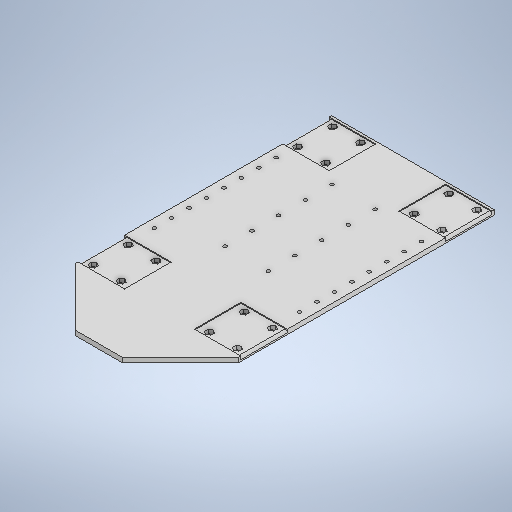
# Autodesk Inventor part: upper_base
Saved by Autodesk Inventor 2025 (Build 290162010, 162A)
## iProperties
Created: 2024-10-24
Part Number: upper_base
Material: Generic
Document SubType Name: Modeling
Designer: fist5
Density: 1 g/cm^3
Appearance: Default
Author: fist5
Autodesk Inventor part; units mm, degrees
ref_plane "YZ Plane" through (0, 0, 0) normal (1, 0, 0) x (0, 1, 0)
ref_plane "XZ Plane" through (0, 0, 0) normal (0, 1, 0) x (-1, 0, 0)
ref_plane "XY Plane" through (0, 0, 0) normal (0, 0, 1) x (1, 0, 0)
sketch "Sketch1" plane through (0, 0, 0) normal (0, 1, 0) x (-1, 0, 0)
  line L0 (-70, 135) -> (-70, -135)
  line L1 (-70, -135) -> (70, -135)
  line L2 (70, -135) -> (70, 135)
  line L3 (70, 135) -> (-70, 135)
  line L4 (-70, 135) -> (70, -135) construction
  line L5 (-70, -135) -> (70, 135) construction
  line L6 (70, 85) -> (20, 135)
  line L7 (-20, 135) -> (-70, 85)
  point P0 (0, 0)
  dimension "d0" = 140
  dimension "d1" = 270
  dimension "d2" = 40
  dimension "d3" = 50
  dimension "d4" = 220
  constraints: 16 end point, 4 point on line, 2 midpoint, 2 parallel, 1 horizontal alignment, 1 perpendicular, 1 vertical
  measures "d0" distance between parallel lines of L0 L2
  measures "d1" distance between parallel lines of L3 L1
  measures "d2" distance of L7.start L6.end
  measures "d3" distance of L6.end L2.end
  measures "d4" distance of L1.end L6.start
extrude "Extrusion1" add sketch "Sketch1" along normal blind 4.05 and the other way blind 4.05 contours L7 L3 L6 L2 L1 L0
sketch "Sketch2" plane through (0, 0, 0) normal (0, 1, 0) x (-1, 0, 0)
  line L0 (70, -135) -> (70, 85) projected
  line L1 (70, 85) -> (20, 135) projected
  line L2 (20, 135) -> (-20, 135) projected
  line L3 (-20, 135) -> (-70, 85) projected
  line L4 (-70, 85) -> (-70, -135) projected
  line L5 (-70, -135) -> (70, -135) projected
  line L6 (70, 83) -> (30, 83)
  line L7 (30, 83) -> (30, 43)
  line L8 (30, 43) -> (70, 43)
  line L9 (70, 43) -> (70, 83)
  line L10 (70, 85) -> (70, -135) projected
  line L11 (70, -133) -> (30, -133)
  line L12 (30, -133) -> (30, -93)
  line L13 (30, -93) -> (70, -93)
  line L14 (70, -93) -> (70, -133)
  line L15 (-30, 43) -> (-30, 83)
  line L16 (-70, 43) -> (-30, 43)
  line L17 (-30, 83) -> (-70, 83)
  line L18 (-70, 83) -> (-70, 43)
  line L19 (-30, -93) -> (-30, -133)
  line L20 (-70, -93) -> (-30, -93)
  line L21 (-30, -133) -> (-70, -133)
  line L22 (-70, -133) -> (-70, -93)
  point P0 (0, 0)
  point P1 (50, 83)
  point P2 (50, -133)
  point P3 (-50, 83)
  point P4 (-50, -133)
  dimension "d11" = 40
  dimension "d12" = 40
  dimension "d13" = 2
  dimension "d14" = 2
  dimension "d15" = 40
  dimension "d16" = 40
  dimension "d19" = 100
  constraints: 32 end point, 4 parallel, 3 horizontal, 2 midpoint, 2 perpendicular, 2 point on line, 18 other
  measures "d11" distance from line of L8 point (50, 83)
  measures "d12" distance between parallel lines of L7 L0
  measures "d13" distance of L6.start L0.end
  measures "d14" distance between parallel lines of L5 L11
  measures "d15" distance between parallel lines of L12 L0
  measures "d16" distance from line of point (50, -133) L13
  measures "d19" distance of L8.end L15.start
extrude "Extrusion2" cut sketch "Sketch2" along normal blind 0.75 and the other way blind 0.75 contours L11 L12 L13 L0 | L4 L20 L19 L21 | L8 L7 L6 L0 | L4 L17 L15 L16
sketch "Sketch3" plane through (0, 0, 0) normal (0, 1, 0) x (-1, 0, 0)
  line L0 (70, -135) -> (70, 85) projected
  line L1 (70, 85) -> (20, 135) projected
  line L2 (20, 135) -> (-20, 135) projected
  line L3 (-20, 135) -> (-70, 85) projected
  line L4 (-70, 85) -> (-70, -135) projected
  line L5 (-70, -135) -> (70, -135) projected
  point P0 (0, 0)
extrude "Extrusion3" cut sketch "Sketch3" along normal up to surface (4.05 mm away)
fillet "Fillet2" radius 2 4 edges at (70, -0.75, 63) (70, -0.75, -113) (-70, -0.75, 63) (-70, -0.75, -113)
sketch "Sketch4" plane through (0, -4.05, 0) normal (0, -1, 0) x (1, 0, 0)
  line L0 (30, -93) -> (70, -93) projected
  line L1 (30, -133) -> (30, -93) projected
  line L2 (70, -133) -> (30, -133) projected
  line L3 (70, -135) -> (70, -133) projected
  line L4 (-70, -135) -> (70, -135) projected
  line L5 (-70, -133) -> (-70, -135) projected
  line L6 (-30, -133) -> (-70, -133) projected
  line L7 (-30, -93) -> (-30, -133) projected
  line L8 (-70, -93) -> (-30, -93) projected
  line L9 (-70, 43) -> (-70, -93) projected
  line L10 (-30, 43) -> (-70, 43) projected
  line L11 (-30, 83) -> (-30, 43) projected
  line L12 (-70, 83) -> (-30, 83) projected
  line L13 (-70, 85) -> (-70, 83) projected
  line L14 (-20, 135) -> (-70, 85) projected
  line L15 (20, 135) -> (-20, 135) projected
  line L16 (70, 85) -> (20, 135) projected
  line L17 (70, 83) -> (70, 85) projected
  line L18 (30, 83) -> (70, 83) projected
  line L19 (30, 43) -> (30, 83) projected
  line L20 (70, 43) -> (30, 43) projected
  line L21 (70, -93) -> (70, 43) projected
  line L22 (62, 78) -> (38, 78)
  line L23 (38, 78) -> (38, 48)
  line L24 (38, 48) -> (62, 48)
  line L25 (62, 48) -> (62, 78)
  line L26 (35.25, 49.5877) -> (38, 51.1754)
  line L27 (38, 51.1754) -> (40.75, 49.5877)
  line L28 (40.75, 49.5877) -> (40.75, 46.4123)
  line L29 (40.75, 46.4123) -> (38, 44.8246)
  line L30 (38, 44.8246) -> (35.25, 46.4123)
  line L31 (35.25, 46.4123) -> (35.25, 49.5877)
  point P0 (0, 0)
  point P1 (35.25, 48)
  dimension "d32" = 24
  dimension "d33" = 30
  dimension "d34" = 5
  dimension "d35" = 8
  dimension "d36" = 5.5
  constraints: 20 end point, 2 parallel, 1 coincident, 1 horizontal, 1 midpoint, 1 perpendicular, 1 point on line, 13 other
  measures "d32" distance between parallel lines of L23 L25
  measures "d33" distance between parallel lines of L24 L22
  measures "d34" distance between parallel lines of L20 L24
  measures "d35" distance between parallel lines of L19 L23
  measures "d36" distance between parallel lines of L31 L28
extrude "Extrusion4" cut sketch "Sketch4" against normal up to surface (4.05 mm away) contours L27 L28 L24 L23 | L23 L24 L28 L29 L30 L31 L26
pattern_linear "Rectangular Pattern1" count 2 spacing 30 along (0, 0, 1) count 2 spacing 24 along (1, 0, 0) of "Extrusion4"
pattern_linear "Rectangular Pattern2" count 2 spacing 176 along (0, 0, -1) count 2 spacing 100 along (-1, 0, 0) of "Extrusion4", "Rectangular Pattern1"
sketch "Sketch6" plane through (0, -4.05, 0) normal (0, -1, 0) x (1, 0, 0)
  line L0 (-70, -135) -> (70, -135) projected
  line L1 (-20, -135) -> (20, -135)
  line L2 (20, -135) -> (20, -132)
  line L3 (20, -132) -> (-20, -132)
  line L4 (-20, -132) -> (-20, -135)
  point P0 (0, 0)
  point P1 (-20, -133.5)
  point P2 (20, -133.5)
  point P3 (0, -135)
  point P4 (20, -135)
  dimension "d51" = 40
  dimension "d52" = 20
  dimension "d53" = 3
  constraints: 8 end point, 3 midpoint, 2 parallel, 1 horizontal, 1 perpendicular, 1 point on line
  measures "d51" distance of point (-20, -133.5) point (20, -133.5)
  measures "d52" distance from line of point (0, -135) L2
  measures "d53" distance between parallel lines of L0 L3
extrude "Extrusion5" add sketch "Sketch6" along normal blind 3
sketch "Sketch7" plane through (0, -4.05, 0) normal (0, -1, 0) x (1, 0, 0)
  line L0 (70, -93) -> (70, 43) projected
  line L1 (70, 13) -> (-70, 13)
  line L2 (-70, 85) -> (-70, -135) projected
  line L3 (20, -135) -> (70, -135) projected
  line L4 (18.5, 8) -> (-18.5, 8)
  line L5 (-18.5, 8) -> (-18.5, -84)
  line L6 (-18.5, -84) -> (18.5, -84)
  line L7 (18.5, -84) -> (18.5, 8)
  line L8 (-20, -132) -> (20, -132) projected
  line L9 (20, -132) -> (-20, -132) projected
  circle A0 centre (18.5, 8) radius 1.5
  point P0 (0, 0)
  point P1 (0, -84)
  point P2 (0, -132)
  point P3 (0, -132)
  dimension "d56" = 148
  dimension "d57" = 5
  dimension "d58" = 37
  dimension "d59" = 92
  dimension "d60" = 3
  constraints: 10 end point, 3 midpoint, 2 horizontal, 2 parallel, 2 point on line, 1 centre point, 1 coincident, 1 perpendicular, 1 vertical alignment
  measures "d56" distance between parallel lines of L3 L1
  measures "d57" distance between parallel lines of L1 L4
  measures "d58" distance between parallel lines of L5 L7
  measures "d59" distance from line of point (0, -84) L4
  measures "d60" diameter of A0
extrude "Extrusion6" cut sketch "Sketch7" against normal up to next contours L7 A0 L4 | L4 A0 L7
pattern_linear "Rectangular Pattern3" count 5 spacing 23 along (0, 0, -1) count 2 spacing 37 along (-1, 0, 0) of "Extrusion6"
sketch "Sketch8" plane through (0, -4.05, 0) normal (0, -1, 0) x (1, 0, 0)
  line L0 (20, -135) -> (70, -135) projected
  line L1 (70, -135) -> (70, 85) projected
  line L2 (-70, -135) -> (-20, -135) projected
  line L3 (-70, 85) -> (-70, -135) projected
  circle A0 centre (62.5, -80) radius 1.5
  circle A1 centre (-62.5, -80) radius 1.5
  point P0 (0, 0)
  dimension "d69" = 55
  dimension "d70" = 7.5
  dimension "d71" = 55
  dimension "d72" = 7.5
  dimension "d73" = 3
  dimension "d74" = 3
  constraints: 2 centre point, 2 coincident
  measures "d69" distance from line of L0 point (62.5, -80)
  measures "d70" distance from line of L1 point (62.5, -80)
  measures "d71" distance from line of L2 point (-62.5, -80)
  measures "d72" distance from line of L3 point (-62.5, -80)
  measures "d73" diameter of A0
  measures "d74" diameter of A1
extrude "Extrusion7" cut sketch "Sketch8" against normal up to next
pattern_linear "Rectangular Pattern4" count 8 spacing 15 along (0, 0, 1) of "Extrusion7"
sketch "Sketch9" plane through (70, 0, -135) normal (0, 0, -1) x (-1, 0, 0)
  line L0 (90, -4.05) -> (87, -4.05) projected
  line L1 (50, -4.05) -> (50, -7.05) projected
  line L2 (90, -4.05) -> (50, -4.05)
  line L3 (50, -4.05) -> (50, -7.05)
  line L4 (50, -7.05) -> (90, -7.05)
  line L5 (90, -7.05) -> (90, -4.05)
  point P0 (70, 0)
  constraints: 8 end point, 2 parallel, 1 horizontal, 1 perpendicular
extrude "Extrusion8" cut sketch "Sketch9" against normal up to next
body "Solid1"
